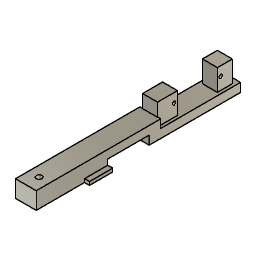
Hotshoe 3 v3 (Autodesk Fusion 360 design; units mm, degrees)
Autodesk Fusion 360 part; units mm, degrees
sketch "hotshoe base" plane through (0, 0, 0) normal (0, 0, 1) x (1, 0, 0)
  line L0 (-100, 65) -> (-87.5, 65)
  line L1 (-87.5, 65) -> (-87.5, 10)
  line L2 (-100, 65) -> (-100, 10)
  line L3 (-100, 10) -> (-87.5, 10)
  line L4 (-87.5, 10) -> (-87.5, -15)
  line L5 (-100, 10) -> (-100, -15)
  line L6 (-100, -14.9671) -> (-87.5, -14.9671)
  line L7 (-87.5, -32.9671) -> (-100, -32.9671)
  line L8 (-100, -32.9671) -> (-100, -58)
  line L9 (-87.5, -32.9671) -> (-87.5, -58)
  line L10 (-87.5, -58) -> (-100, -58)
  line L11 (-100, -30) -> (-100, -19)
  line L12 (-100, -30) -> (-100, -31)
  line L13 (-100, -19) -> (-100, -17)
  line L14 (-100, -15) -> (-100, -17)
  line L15 (-87.5, -15) -> (-87.5, -31)
  line L16 (-100, 10) -> (-100, 17)
  line L17 (-100, 17) -> (-87.5, 17)
  line L18 (-100, -31) -> (-100, -32.9671)
  line L19 (-87.5, -31) -> (-87.5, -33)
  line L20 (-87.5, -15) -> (-87.5, -14.9328)
  line L21 (-100, -15) -> (-103, -15)
  line L22 (-87.5, -14.9328) -> (-84.5, -14.9328)
  line L23 (-103, -15) -> (-103, -29)
  line L24 (-103, -29) -> (-100, -29)
  line L25 (-84.5, -14.9328) -> (-84.5, -28.9328)
  line L26 (-84.5, -28.9328) -> (-87.5, -28.9328)
  dimension "d1" = 12.5
  dimension "d2" = 55
  dimension "d3" = 55
  dimension "d4" = 25
  dimension "d7" = 43
  dimension "d8" = 43
  dimension "d12" = 7
  dimension "d102" = 3
  dimension "d103" = 3
  dimension "d107" = 14
  dimension "d108" = 14
  constraint horizontal L0
  constraint perpendicular L0 L1
  constraint perpendicular L0 L2
  constraint perpendicular L3 L4
  constraint perpendicular L3 L5
  constraint perpendicular L5 L6
  constraint perpendicular L7 L8
  constraint perpendicular L3 L16
  constraint coincident L1 L17.end
  constraint perpendicular L1 L17
  constraint coincident L9 L19.end
  constraint perpendicular L7 L19
  constraint coincident L4 L20.end
  constraint coincident L5 L6.start
  constraint coincident L4 L6.end
  constraint perpendicular L14 L21
  constraint perpendicular L15 L22
  constraint perpendicular L21 L23
  constraint coincident L11 L24.end
  constraint perpendicular L11 L24
  constraint perpendicular L22 L25
  constraint coincident L15 L26.end
  constraint perpendicular L15 L26
  measures "d1" distance of L0.start L0.end
  measures "d2" distance of L0.end L1.end
  measures "d3" distance of L0.start L2.end
  measures "d4" distance of L1.end L4.end
  measures "d7" distance of L5.end L8.end
  measures "d8" distance of L4.end L9.end
  measures "d12" distance of L2.end L16.end
  measures "d102" distance of L5.end L21.end
  measures "d103" distance of L20.end L22.end
  measures "d107" distance of L21.end L23.end
  measures "d108" distance of L22.end L25.end
combine "Combine1" [no effect]
combine "Combine2" [no effect]
move_body "Move1" [no effect]
move_body "Move2" [no effect]
combine "Combine3" [no effect]
combine "Combine4" [no effect]
sketch "servo attachment " plane through (0, 0, 5.25) normal (0, 0, 1) x (-1, 0, 0)
  line L0 (100, -17.1) -> (87.5, -17.1)
  line L1 (87.5, -17.1) -> (87.5, -65.1)
  line L2 (87.5, -65.1) -> (100, -65.1)
  line L3 (100, -65.1) -> (100, -17.1)
  line L4 (65.1287, -21.8482) -> (74.1287, -21.8482)
  line L5 (74.1287, -21.8482) -> (74.1287, -45.8482)
  line L6 (65.1287, -21.8482) -> (65.1287, -45.8482)
  line L7 (65.1287, -45.8482) -> (74.1287, -45.8482)
  line L8 (74.1287, -21.8482) -> (74.1287, -9.8482)
  line L9 (65.1287, -21.8482) -> (65.1287, -9.8482)
  line L10 (65.1287, -9.8482) -> (74.1287, -9.8482)
  line L11 (74.1287, -45.8482) -> (74.1287, -54.8482)
  line L12 (65.1287, -45.8482) -> (65.1287, -54.8482)
  line L13 (65.1287, -54.8482) -> (74.1287, -54.8482)
  dimension "d39" = 9
  dimension "d40" = 24
  dimension "d41" = 24
  dimension "d42" = 12
  dimension "d43" = 9
  dimension "d44" = 9
  constraint horizontal L4
  constraint perpendicular L4 L5
  constraint perpendicular L4 L6
  constraint perpendicular L5 L7
  constraint perpendicular L4 L8
  constraint perpendicular L4 L9
  constraint perpendicular L8 L10
  constraint perpendicular L7 L11
  constraint perpendicular L7 L12
  constraint perpendicular L11 L13
  measures "d39" distance of L4.start L4.end
  measures "d40" distance of L4.end L5.end
  measures "d41" distance of L4.start L6.end
  measures "d42" distance of L4.end L8.end
  measures "d43" distance of L5.end L11.end
  measures "d44" distance of L6.end L12.end
sketch "servo screw holes" plane through (-74.1287, 0, 0) normal (-1, 0, 0) x (0, -1, 0)
  line L0 (-54.8482, 5.25) -> (-45.8482, 5.25)
  line L1 (-45.8482, 5.25) -> (-45.8482, 20.25)
  line L2 (-45.8482, 20.25) -> (-54.8482, 20.25)
  line L3 (-54.8482, 20.25) -> (-54.8482, 5.25)
  circle A0 centre (-47.8482, 12.75) radius 1
  circle A1 centre (-19.7934, 12.75) radius 1
  dimension "d54" = 2
  dimension "d55" = 2
  measures "d54" diameter of A0
  measures "d55" diameter of A1
combine "Combine5" [no effect]
move_body "Move4" [no effect]
move_body "Move5" [no effect]
move_body "Move6" [no effect]
move_body "Move7" [no effect]
combine "Combine6" [no effect]
sketch "screw hole for counter weight" plane through (0, 0, 0) normal (0, 0, 1) x (1, 0, 0)
  circle A0 centre (-93.75, -50) radius 1.7
  dimension "d97" = 3.4
  measures "d97" diameter of A0
extrude "Extrude29" add sketch "hotshoe base" along normal blind 10.25 contours L4 L5 L6 L7 L11 L12 L13 L14 L15 L18 L19 L20 | L7 L8 L9 L10 L19 makes body 1
extrude "Extrude30" add sketch "hotshoe base" along normal blind 5.25 contours L3 L4 L5 L6 L20 bodies 1
extrude "Extrude31" add 1 faces at (-95.8333, 1.6776, 5.25) along direction (0, 0, 1) blind 5 on bodies 1 bodies 1
extrude "Extrude32" cut sketch "hotshoe base" along normal blind 5.25 contours L3 L4 L5 L6 L20 bodies 1
extrude "Extrude33" add sketch "hotshoe base" along normal blind 10.25 contours L1 L2 L3 L16 L17 bodies 1
extrude "Extrude34" add sketch "hotshoe base" along normal blind 5.25 contours L0 L1 L2 L17 bodies 1
extrude "Extrude35" add sketch "hotshoe base" along normal blind 2 contours L11 L13 L14 L21 L23 L24 bodies 1
extrude "Extrude36" add sketch "hotshoe base" along normal blind 2 contours L4 L15 L20 L22 L25 L26 bodies 1
extrude "Extrude37" cut sketch "screw hole for counter weight" along normal blind 23 bodies 1
extrude "Extrude38" add sketch "servo attachment " along normal blind 13 separate body contours L4 L8 L9 L10 makes body 2
extrude "Extrude39" add sketch "servo attachment " along normal blind 13 separate body contours L7 L11 L12 L13 makes body 3
extrude "Extrude40" cut sketch "servo screw holes" against normal blind 15 contours A0 | A1 bodies 2 3
move_body "Move14" bodies 2 3 to x (1, 0, 0) y (0, 1, 0) z (0, 0, 1) at (-24.1244, 7.0601, 0.053)
move_body "Move15" bodies 3 2 to x (1, 0, 0) y (0, 1, 0) z (0, 0, 1) at (0, -0.1052, -0.1477)
combine "Combine7" operation add target body 1 tool bodies 3 2
named bodies: "hotshoe"
